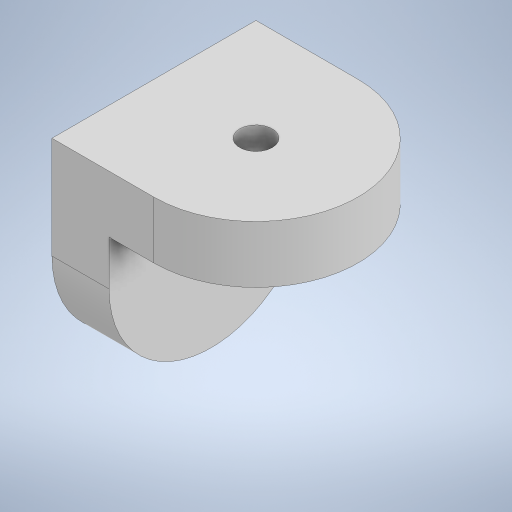
# Autodesk Inventor part: Frame Connector
Saved by Autodesk Inventor 2024 (Build 280153000, 153)
## iProperties
Created: 2024-03-09
Part Number: Frame Connector
Material: Generic
Document SubType Name: Modeling
Designer: ddcos
Density: 1 g/cm^3
Appearance: Default
Author: ddcos
Autodesk Inventor part; units mm, degrees
ref_plane "YZ Plane" through (0, 0, 0) normal (1, 0, 0) x (0, 1, 0)
ref_plane "XZ Plane" through (0, 0, 0) normal (0, 1, 0) x (-1, 0, 0)
ref_plane "XY Plane" through (0, 0, 0) normal (0, 0, 1) x (1, 0, 0)
sketch "Sketch1" plane through (0, 0, 0) normal (0, 0, 1) x (1, 0, 0)
  line L0 (0, 0) -> (-25, 0)
  line L1 (-25, 0) -> (-25, 25)
  line L2 (-25, 25) -> (0, 25)
  line L3 (0, 25) -> (0, 0)
  dimension "d0" = 25
  dimension "d1" = 25
  constraints: 8 end point, 2 parallel, 1 horizontal, 1 perpendicular
  measures "d0" distance of L2.end L0.start
  measures "d1" distance of L0.start L0.end
extrude "Extrusion1" add sketch "Sketch1" along normal blind 25
sketch "Sketch2" plane through (-25, 25, 0) normal (0, 1, 0) x (1, 0, 0)
  circle A0 centre (12.5, -12.5) radius 2
  line L0 (25, 0) -> (25, -25) projected
  line L1 (25, 0) -> (0, 0) projected
  arc A1 (12.5, -25) -> (12.5, 0) centre (12.5, -12.5) ccw
  line L2 (25, -25) -> (0, -25) projected
  point P0 (25, -12.5)
  dimension "d4" = 4
  dimension "d5" = 12.5
  dimension "d6" = 12.5
  constraints: 2 centre point, 2 point on circle, 1 midpoint, 1 tangent
  measures "d4" diameter of A0
  measures "d5" distance from line of L0 A0.centre
  measures "d6" distance from line of L1 A0.centre
extrude "Extrusion2" cut sketch "Sketch2" against normal blind 25
sketch "Sketch3" plane through (0, 0, 25) normal (0, 0, 1) x (1, 0, 0)
  line L0 (0, 0) -> (-18, 0)
  line L1 (-18, 0) -> (-18, 18)
  line L2 (-18, 18) -> (0, 18)
  line L3 (0, 18) -> (0, 0)
  dimension "d9" = 18
  dimension "d10" = 18
  constraints: 8 end point, 2 parallel, 1 horizontal, 1 perpendicular
  measures "d9" distance of L1.end L2.end
  measures "d10" distance of L0.end L1.end
extrude "Extrusion3" cut sketch "Sketch3" against normal blind 25
sketch "Sketch4" plane through (-18, 0, 25) normal (1, 0, 0) x (0, 0, -1)
  circle A0 centre (12.5, 12.5) radius 2
  line L0 (25, 0) -> (0, 0) projected
  line L1 (25, 18) -> (25, 0) projected
  arc A1 (0, 12.5) -> (25, 12.5) centre (12.5, 12.5) ccw
  line L2 (0, 0) -> (0, 18) projected
  point P0 (12.5, 0)
  dimension "d13" = 4
  dimension "d14" = 12.5
  dimension "d15" = 12.5
  constraints: 2 centre point, 2 point on circle, 1 point on line, 1 tangent
  measures "d13" diameter of A0
  measures "d14" distance from line of L0 A0.centre
  measures "d15" distance from line of L1 A0.centre
extrude "Extrusion4" cut sketch "Sketch4" against normal blind 25
body "Solid1"
